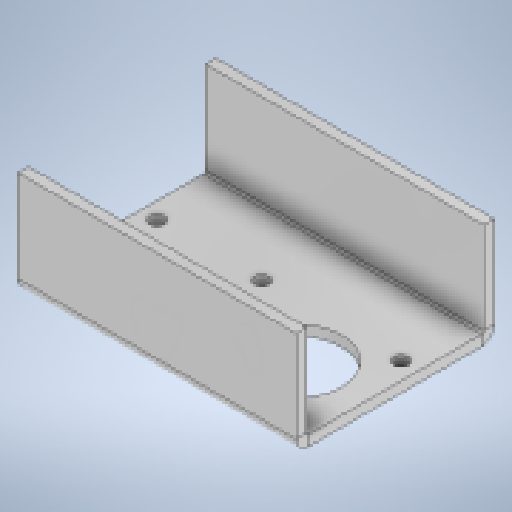
# Autodesk Inventor part: body_motor_frame
Saved by Autodesk Inventor 2025.2 (Build 292293000, 293)
## iProperties
Created: 2025-05-07
Part Number: body_motor_frame
Material: Aluminum 6061-AHC
Document SubType Name: Sheet Metal
Designer: chris
Density: 2.7 g/cm^3
Sheet Metal Rule: Default_mm
Appearance: Aluminum - Dark
Author: chris
Autodesk Inventor part; units mm, degrees
ref_plane "YZ Plane" through (0, 0, 0) normal (1, 0, 0) x (0, 1, 0)
ref_plane "XZ Plane" through (0, 0, 0) normal (0, 1, 0) x (-1, 0, 0)
ref_plane "XY Plane" through (0, 0, 0) normal (0, 0, 1) x (1, 0, 0)
sketch "Sketch1" plane through (0, 0, 0) normal (0, 1, 0) x (-1, 0, 0)
  line L0 (0, 0) -> (40, 0)
  line L1 (40, 0) -> (40, -28.5)
  line L2 (40, -28.5) -> (0, -28.5)
  line L3 (0, -28.5) -> (0, 0)
  dimension "d0" = 40
  dimension "d1" = 28.5
  measures "d0" distance of L1.end L2.end
  measures "d1" distance of L0.end L1.end
extrude "Plate1" add sketch "Sketch1" along normal blind 1.5
sketch "Sketch2" plane through (0, 0, -1.5) normal (0, 0, 1) x (1, 0, 0)
  line L0 (-40, 0) -> (0, 0)
  line L1 (0, 0) -> (0, 15)
  line L2 (0, 15) -> (-40, 15)
  line L3 (-40, 15) -> (-40, 0)
  constraints: 6 end point, 1 horizontal, 1 perpendicular, 1 vertical
edge flange "Flange1" height 15 angle 90 thickness 1.5 bend radius 0.31 thickness toward (0, 0, 1) relief straight relief width 1.5 relief depth 0.75 edges at (-20, 1.5, 0) wall of the first edge with corners at (-40, 0, -1.5) (0, 0, -1.5) (0, 15, -1.5) (-40, 15, -1.5)
bend "Bend1"
corner "Corner1"
sketch "Sketch3" plane through (-40, 0, -27) normal (0, 0, -1) x (-1, 0, 0)
  line L0 (-40, 0) -> (0, 0)
  line L1 (0, 0) -> (0, 15)
  line L2 (0, 15) -> (-40, 15)
  line L3 (-40, 15) -> (-40, 0)
  constraints: 6 end point, 1 horizontal, 1 perpendicular, 1 vertical
edge flange "Flange2" height 15 angle 90 thickness 1.5 bend radius 0.31 thickness toward (0, 0, -1) relief straight relief width 1.5 relief depth 0.75 edges at (-20, 1.5, -28.5) wall of the first edge with corners at (0, 0, -27) (-40, 0, -27) (-40, 15, -27) (0, 15, -27)
bend "Bend2"
corner "Corner2"
sketch "Sketch4" plane through (0, 0, 0) normal (0, -1, 0) x (1, 0, 0)
  ellipse E0 centre (-2.118, -4.118) end of major axis (-1.252, -3.252) minor radius 1 (-1, -3.8944) -> (-1.8944, -3) ccw projected
  line L0 (-1, -20.2456) -> (-1, -3.8944) projected
  ellipse E1 centre (-2.118, -20.022) end of major axis (-1.252, -20.888) minor radius 1 (-1.8944, -21.14) -> (-1, -20.2456) ccw projected
  line L1 (-38.2056, -21.14) -> (-1.8944, -21.14) projected
  ellipse E2 centre (-37.982, -20.022) end of major axis (-38.848, -20.888) minor radius 1 (-39.1, -20.2456) -> (-38.2056, -21.14) ccw projected
  line L2 (-39.1, -3.8944) -> (-39.1, -20.2456) projected
  ellipse E3 centre (-37.982, -4.118) end of major axis (-38.848, -3.252) minor radius 1 (-38.2056, -3) -> (-39.1, -3.8944) ccw projected
  line L3 (-1.8944, -3) -> (-38.2056, -3) projected
  circle A0 centre (-37.6, -19.595) radius 0.7835 projected
  circle A1 centre (-37.6, -4.545) radius 0.7835 projected
  circle A2 centre (-22.5, -19.595) radius 0.7835 projected
  circle A3 centre (-22.5, -4.545) radius 0.7835 projected
  circle A4 centre (-2.5, -19.595) radius 0.7835 projected
  circle A5 centre (-2.5, -4.545) radius 0.7835 projected
  circle A6 centre (-10, -12.07) radius 6.4 projected
  point P0 (0, 0)
  constraints: 4 other
hole "Hole1" at (-2.5, 0, -19.595) at (-2.5, 0, -4.545) at (-22.5, 0, -19.595) at (-22.5, 0, -4.545) at (-37.6, 0, -19.595) at (-37.6, 0, -4.545) direction (0, 1, 0) diameter 2.1 depth 1.5
equation "\"d28\" = Thickness"
equation "\"d2\" = Thickness"
equation "\"d3\" = BendReliefWidth"
equation "\"d4\" = BendReliefDepth"
equation "\"d5\" = MinimumRemnant"
equation "\"d6\" = TransitionRadius"
equation "\"d9\" = BendRadius"
equation "\"d10\" = CornerReliefSize"
equation "\"d11\" = GapSize"
equation "\"d12\" = JacobiRadiusSize"
equation "\"d13\" = BendReliefWidth"
equation "\"d14\" = BendReliefDepth"
equation "\"d15\" = MinimumRemnant"
equation "\"d16\" = TransitionRadius"
equation "\"d19\" = BendRadius"
equation "\"d20\" = CornerReliefSize"
equation "\"d21\" = GapSize"
equation "\"d22\" = JacobiRadiusSize"
equation "\"BendReliefWidth\" = Thickness"
equation "\"BendReliefDepth\" = 0.5 * Thickness"
equation "\"CornerReliefSize\" = 4 * Thickness"
equation "\"MinimumRemnant\" = 2 * Thickness"
equation "\"TransitionRadius\" = BendRadius"
equation "\"JacobiRadiusSize\" = BendRadius"
equation "\"GapSize\" = Thickness"
equation "\"Thickness\" = 1.5"
equation "\"BendRadius\" = 0.31"
body "Solid1"
